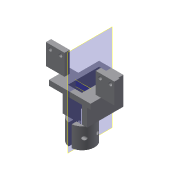
# Autodesk Inventor part: servoplace
Saved by Autodesk Inventor 2018 (Build 220112000, 112)
## iProperties
Created: 2018-08-06
Part Number: servoplace
Material: Generic
Document SubType Name: Sheet Metal
Designer: Bardo91
Density: 1 g/cm^3
Sheet Metal Rule: Default_mm
Appearance: Default
Author: Bardo91
Autodesk Inventor part; units mm, degrees
note: some values were not read from the file. Chosen so that the rebuilt part matches the saved one: sketch regions of "Extrusion1".
ref_plane "YZ Plane" through (0, 0, 0) normal (1, 0, 0) x (0, 1, 0)
ref_plane "XZ Plane" through (0, 0, 0) normal (0, 1, 0) x (-1, 0, 0)
ref_plane "XY Plane" through (0, 0, 0) normal (0, 0, 1) x (1, 0, 0)
sketch "Sketch1" plane through (0, 0, 0) normal (0, 0, 1) x (1, 0, 0)
  line L0 (0, 0) -> (13.5, 0)
  line L1 (13.5, 0) -> (13.5, 30)
  line L2 (13.5, 30) -> (0, 30)
  line L3 (0, 30) -> (0, 0)
  line L4 (-5, 35) -> (18.5, 35)
  line L5 (18.5, 35) -> (18.5, -5)
  line L6 (18.5, -5) -> (-5, -5)
  line L7 (-5, -5) -> (-5, 35)
  line L8 (6.75, -5) -> (-13.25, -5)
  line L9 (-13.25, -5) -> (-13.25, 15)
  line L10 (-13.25, 15) -> (-5, 15)
  line L11 (6.75, -5) -> (26.75, -5)
  line L12 (26.75, -5) -> (26.75, 15)
  line L13 (26.75, 15) -> (18.5, 15)
  dimension "d0" = 13.5
  dimension "d1" = 30
  dimension "d2" = 5
  dimension "d5" = 20
  dimension "d6" = 20
  dimension "d7" = 20
  dimension "d8" = 20
  constraints: 28 end point, 7 perpendicular, 4 point on line, 3 midpoint, 2 horizontal, 3 other
  measures "d0" distance of L0.start L0.end
  measures "d1" distance of L0.end L1.end
  measures "d2" distance between parallel lines of L2 L4
  measures "d5" distance of L8.start L8.end
  measures "d6" distance of L8.end L9.end
  measures "d7" distance of L8.start L11.end
  measures "d8" distance of L11.end L12.end
extrude "Extrusion1" add sketch "Sketch1" along normal blind 5
sketch "Sketch10" plane through (0, 0, 0) normal (0, 0, -1) x (-1, 0, 0)
  line L0 (-13.5, 30) -> (-13.5, 0) projected
  line L1 (-13.5, 0) -> (-18.5, 0)
  line L2 (-18.5, 0) -> (-18.5, 35)
  line L3 (-18.5, 35) -> (-13.5, 35)
  line L4 (-13.5, 35) -> (-13.5, 0)
  line L5 (0, 0) -> (0, 30) projected
  line L6 (5, 35) -> (5, 15) projected
  line L7 (0, 0) -> (5, 0)
  line L8 (5, 0) -> (5, 35)
  line L9 (5, 35) -> (0, 35)
  line L10 (0, 35) -> (0, 0)
  constraints: 16 end point, 4 parallel, 2 horizontal, 2 perpendicular
extrude "Extrusion10" add sketch "Sketch10" along normal blind 21.5
sketch "Sketch11" plane through (0, 0, -21.5) normal (0, 0, -1) x (-1, 0, 0)
  line L0 (-13.5, 30) -> (-13.5, 0) projected
  line L1 (-13.5, 0) -> (-13.5, 7)
  line L2 (-18.5, 35) -> (-18.5, 0) projected
  line L3 (-6.75, 7) -> (-6.75, 13)
  line L4 (-6.75, 13) -> (-16.8526, 13)
  line L5 (-6.75, 13) -> (3.3526, 13)
  line L6 (-6.75, 13) -> (-8.25, 13)
  line L7 (-6.75, 13) -> (-5.25, 13)
  arc A0 (-16.8526, 13) -> (-8.25, -4.6539) centre (-6.75, 7) ccw
  arc A1 (-5.25, -4.6539) -> (3.3526, 13) centre (-6.75, 7) ccw
  arc A2 (-5.25, 5) -> (-6.75, 9.5) centre (-6.75, 7) ccw
  arc A3 (-8.25, 9) -> (-8.25, 5) centre (-6.75, 7) ccw
  line L8 (-5.25, 13) -> (-5.25, 9)
  line L9 (-5.25, 7) -> (-5.25, -4.6539)
  line L10 (-8.25, 13) -> (-8.25, 9)
  line L11 (-8.25, 7) -> (-8.25, -4.6539)
  line L12 (-13.5, 7) -> (-8.25, 7)
  line L13 (-5.25, 7) -> (0, 7)
  point P0 (0, 0)
  dimension "d45" = 7
  dimension "d47" = 6
  dimension "d48" = 1.5
  dimension "d49" = 1.5
  constraints: 24 end point, 9 point on circle, 7 perpendicular, 7 point on line, 4 centre point, 1 coincident, 1 tangent, 1 vertical
  measures "d45" distance of L0.end L1.end
  measures "d47" distance of L3.start L3.end
  measures "d48" distance of L3.end L6.end
  measures "d49" distance of L3.end L7.end
extrude "Extrusion11" add sketch "Sketch11" along normal blind 20 contours L4 L10 A3 L12 L0 | L0 L12 A3 L11 A0 L4 | L8 L5 A1 L9 A2
sketch "Sketch12" plane through (18.5, 15, 5) normal (1, 0, 0) x (0, 0, -1)
  line L0 (26.5, -2) -> (26.5, -6) projected
  line L1 (26.5, -10) -> (46.5, -10) projected
  line L2 (26.5, -6) -> (26.5, -10)
  line L3 (26.5, -15) -> (26.5, -8) projected
  line L4 (26.5, -10) -> (26.5, -8)
  line L5 (26.5, -8) -> (46.4389, -8)
  line L6 (36.4695, -8) -> (36.4695, -15)
  line L7 (36.4695, -8) -> (36.4695, -2)
  line L8 (36.4695, -8) -> (42.4695, -8) construction
  line L9 (36.4695, -2) -> (36.4695, -4)
  circle A0 centre (36.4695, -4) radius 1.75
  circle A1 centre (36.4695, -15) radius 1.75
  point P0 (5, -15)
  dimension "d52" = 90
  dimension "d53" = 2
  dimension "d54" = 3.5
  dimension "d55" = 3.5
  constraints: 14 end point, 3 perpendicular, 2 centre point, 2 coincident, 1 collinear, 1 horizontal, 1 midpoint, 1 point on line, 1 vertical
  measures "d52" angle of L8 L7
  measures "d53" distance of L7.end L9.end
  measures "d54" diameter of A0
  measures "d55" diameter of A1
extrude "Extrusion12" cut sketch "Sketch12" against normal through all contours A0 L7 | L7 A0 | A1
sketch "Sketch13" plane through (13.5, 0, 5) normal (-1, 0, 0) x (0, 0, 1)
  line L0 (-26.5, 13) -> (-46.5, 13) projected
  line L1 (-26.5, 13) -> (-26.5, 0)
  line L2 (-26.5, 0) -> (-39.5, 13)
  line L3 (-39.5, 13) -> (-26.5, 13)
  point P0 (-5, 0)
  dimension "d64" = 45
  constraints: 6 end point, 1 collinear, 1 point on line, 1 vertical
  measures "d64" angle of L1 L2
extrude "Extrusion13" cut sketch "Sketch13" along normal up to surface (13.5 mm away)
ref_plane "Work Plane1" through (0, 7.5, 5) normal (0, 1, 0) x (1, 0, 0)
sketch "Sketch16" plane through (0, 7.5, 5) normal (0, 1, 0) x (1, 0, 0)
  line L0 (-13.25, 5) -> (-13.25, 0) projected
  line L1 (-13.25, 0) -> (-8.25, 0)
  line L2 (-13.25, 0) -> (26.75, 0) projected
  line L3 (-8.25, 0) -> (-8.25, -5)
  line L4 (-8.25, -5) -> (-8.25, -5)
  line L5 (-8.25, -5) -> (-8.25, -15)
  line L6 (-8.25, -15) -> (-26.25, -15)
  line L7 (-26.25, -15) -> (-26.25, 0)
  line L8 (-26.25, 0) -> (-13.25, 0)
  line L9 (-8.25, -15) -> (-8.25, -11)
  line L10 (-8.25, -11) -> (-12.25, -11)
  line L11 (-12.25, -11) -> (-22.25, -11)
  circle A0 centre (-12.25, -11) radius 1.75
  circle A1 centre (-22.25, -11) radius 1.75
  point P0 (0, 5)
  dimension "d88" = 5
  dimension "d89" = 5
  dimension "d90" = 0
  dimension "d91" = 10
  dimension "d92" = 18
  dimension "d93" = 4
  dimension "d94" = 4
  dimension "d95" = 10
  dimension "d96" = 3.5
  dimension "d97" = 3.5
  constraints: 20 end point, 7 perpendicular, 4 point on line, 2 centre point, 2 coincident
  measures "d88" distance of L0.end L1.end
  measures "d89" distance of L1.end L3.end
  measures "d90" distance of L3.end L4.end
  measures "d91" distance of L4.end L5.end
  measures "d92" distance of L5.end L6.end
  measures "d93" distance of L5.end L9.end
  measures "d94" distance of L9.end L10.end
  measures "d95" distance of L10.end L11.end
  measures "d96" diameter of A0
  measures "d97" diameter of A1
extrude "Extrusion16" add sketch "Sketch16" along normal mid plane 5
ref_plane "Work Plane2" through (6.75, 0, 5) normal (-1, 0, 0) x (0, 0, 1)
mirror "Mirror1" about plane through (6.75, 0, 5) normal (-1, 0, 0) of "Extrusion16"
fillet "Fillet1" radius 2 1 edges at (6.75, 30, 0)
equation "\"BendRadius\" = Thickness"
equation "\"BendReliefWidth\" = Thickness"
equation "\"BendReliefDepth\" = 0.5 * Thickness"
equation "\"CornerReliefSize\" = 4 * Thickness"
equation "\"MinimumRemnant\" = 2 * Thickness"
equation "\"TransitionRadius\" = BendRadius"
equation "\"JacobiRadiusSize\" = BendRadius"
equation "\"GapSize\" = Thickness"
equation "\"Thickness\" = 0.5"
body "Solid1"
